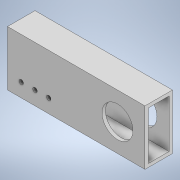
# Autodesk Inventor part: Intake mount
Saved by Autodesk Inventor 2022 (Build 260153000, 153)
## iProperties
Created: 2023-01-17
Part Number: Intake mount
Material: Generic
Document SubType Name: Modeling
Designer: s135320
Density: 1 g/cm^3
Appearance: Default
Author: s135320
Autodesk Inventor part; units mm, degrees
ref_plane "YZ Plane" through (0, 0, 0) normal (1, 0, 0) x (0, 1, 0)
ref_plane "XZ Plane" through (0, 0, 0) normal (0, 1, 0) x (-1, 0, 0)
ref_plane "XY Plane" through (0, 0, 0) normal (0, 0, 1) x (1, 0, 0)
sketch "Sketch1" plane through (0, 0, 0) normal (0, 0, 1) x (1, 0, 0)
  line L0 (0, 0) -> (127, 0)
  line L1 (127, 0) -> (127, 50.8)
  line L2 (127, 50.8) -> (0, 50.8)
  line L3 (0, 50.8) -> (0, 0)
  dimension "d0" = 50.8
  dimension "d1" = 127
  constraints: 8 end point, 2 parallel, 1 horizontal, 1 perpendicular
  measures "d0" distance of L2.end L0.start
  measures "d1" distance of L0.start L0.end
extrude "Extrusion1" add sketch "Sketch1" along normal blind 25.4
shell "Shell1" thickness 3.175 removed faces 2 at (0, 33.8667, 16.9333) at (127, 16.9333, 8.4667)
sketch "Sketch2" plane through (0, 0, 25.4) normal (0, 0, 1) x (1, 0, 0)
  line L0 (0, 3.175) -> (0, 47.625) projected
  line L1 (0, 25.4) -> (101.6, 25.4)
  circle A0 centre (101.6, 25.4) radius 14.2875
  line L2 (127, 0) -> (127, 50.8) projected
  point P0 (0, 0)
  dimension "d5" = 28.575
  dimension "d9" = 25.4
  constraints: 2 end point, 1 centre point, 1 coincident, 1 horizontal, 1 midpoint
  measures "d5" diameter of A0
  measures "d9" distance from line of L2 L1.end
extrude "Extrusion2" cut sketch "Sketch2" against normal through all
sketch "Sketch3" plane through (0, 0, 25.4) normal (0, 0, 1) x (1, 0, 0)
  line L0 (0, 50.8) -> (0, 12.7)
  line L1 (0, 3.175) -> (0, 47.625) projected
  line L2 (0, 12.7) -> (12.7, 12.7)
  circle A0 centre (12.7, 12.7) radius 2.0701
  circle A1 centre (25.4, 12.7) radius 2.0701
  circle A2 centre (38.1, 12.7) radius 2.0701
  point P0 (0, 0)
  dimension "d12" = 12.7
  dimension "d13" = 4.1402
  dimension "d16" = 12.7
  dimension "d23" = 12.7
  constraints: 4 end point, 3 centre point, 2 horizontal, 1 coincident, 1 point on line, 4 other
  measures "d12" distance of L0.end L2.end
  measures "d13" diameter of A0
  measures "d16" distance of A0.centre A1.centre
  measures "d23" distance of point (0, 0) L0.end
extrude "Extrusion3" cut sketch "Sketch3" against normal through all
body "Solid1"
